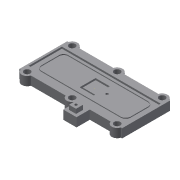
# Autodesk Inventor part: Bottom 6_12
Saved by Autodesk Inventor 2016 (Build 200138000, 138)
## iProperties
Created: 2015-05-18
Part Number: Bottom 6_12
Material: Generic
Document SubType Name: Modeling
Designer: Jonathan
Density: 1 g/cm^3
Appearance: Default
Author: Jonathan
Autodesk Inventor part; units mm, degrees
ref_plane "YZ Plane" through (0, 0, 0) normal (1, 0, 0) x (0, 1, 0)
ref_plane "XZ Plane" through (0, 0, 0) normal (0, 1, 0) x (-1, 0, 0)
ref_plane "XY Plane" through (0, 0, 0) normal (0, 0, 1) x (1, 0, 0)
sketch "Sketch1" plane through (0, 0, 0) normal (0, 1, 0) x (-1, 0, 0)
  line L0 (58, 27) -> (-58, 27)
  line L1 (-58, 27) -> (-58, -27)
  line L2 (-58, -27) -> (58, -27)
  line L3 (58, -27) -> (58, 27)
  line L4 (58, 27) -> (-58, -27) construction
  line L5 (-58, 27) -> (58, -27) construction
  point P0 (0, 0)
  dimension "d0" = 116
  dimension "d1" = 54
  constraints: 12 end point, 2 midpoint, 2 parallel, 1 horizontal, 1 perpendicular
  measures "d0" distance of L2.end L1.end
  measures "d1" distance of L2.end L0.start
extrude "Body" add sketch "Sketch1" along normal mid plane 10
sketch "Sketch2" plane through (0, 5, 0) normal (0, 1, 0) x (1, 0, 0)
  line L0 (-55.75, 18.75) -> (55.75, 18.75)
  line L1 (55.75, 18.75) -> (55.75, -18.75)
  line L2 (55.75, -18.75) -> (-55.75, -18.75)
  line L3 (-55.75, -18.75) -> (-55.75, 18.75)
  line L4 (-55.75, 18.75) -> (55.75, -18.75) construction
  line L5 (55.75, 18.75) -> (-55.75, -18.75) construction
  point P0 (0, 0)
  dimension "d4" = 111.5
  dimension "d5" = 37.5
  constraints: 12 end point, 2 midpoint, 2 parallel, 1 horizontal, 1 perpendicular
  measures "d4" distance of L1.end L2.end
  measures "d5" distance of L0.end L1.end
extrude "Top Socket" cut sketch "Sketch2" against normal blind 2
sketch "Sketch3" plane through (0, 3, 0) normal (0, 1, 0) x (1, 0, 0)
  line L0 (-8, -9) -> (8, -9)
  line L1 (8, -9) -> (8, 9)
  line L2 (8, 9) -> (-8, 9)
  line L3 (-8, 9) -> (-8, -9)
  line L4 (-8, -9) -> (8, 9) construction
  line L5 (8, -9) -> (-8, 9) construction
  point P0 (0, 0)
  dimension "d29" = 18
  dimension "d30" = 16
  constraints: 12 end point, 2 midpoint, 2 parallel, 1 horizontal, 1 perpendicular
  measures "d29" distance of L2.end L0.start
  measures "d30" distance of L1.end L2.end
extrude "Photoelectrode Bay" cut sketch "Sketch3" against normal blind 2
sketch "Sketch4" plane through (0, 3, 0) normal (0, 1, 0) x (1, 0, 0)
  circle A0 centre (14, 0) radius 1.45
  line L0 (-55.75, -18.75) -> (-55.75, 18.75) projected
  line L1 (-55.75, 0) -> (55.75, 0)
  line L2 (55.75, 18.75) -> (55.75, -18.75) projected
  line L3 (-55.75, -3) -> (55.75, -3)
  line L4 (8, 9) -> (8, -9) projected
  point P0 (0, 0)
  dimension "d11" = 2.9
  dimension "d20" = 3
  dimension "d97" = 6
  constraints: 4 end point, 2 midpoint, 2 point on line, 1 centre point, 1 parallel
  measures "d11" diameter of A0
  measures "d20" distance between parallel lines of L1 L3
  measures "d97" distance from line of A0.centre L4
revolve "Ref elec" cut sketch "Sketch4" angle 90 about axis through (-55.75, 3, 3) along (-1, 0, 0) contours L1 A0 | A0 L1
sketch "Sketch7" plane through (-58, 5, 27) normal (0, 0, 1) x (1, 0, 0)
  circle A0 centre (72, -5) radius 1.45
  circle A1 centre (72, -5) radius 1.45 projected
  point P0 (58, -5)
  dimension "d21" = 2.9
  constraints: 1 centre point, 1 concentric
  measures "d21" diameter of A0
extrude "Ref elec length" cut sketch "Sketch7" against normal up to surface (24 mm away)
sketch "Sketch8" plane through (-58, 5, 27) normal (0, 0, 1) x (1, 0, 0)
  line L0 (116, -10) -> (0, -10) projected
  line L1 (113.75, 0) -> (2.25, 0) projected
  line L2 (64.5, 0) -> (79.5, 0)
  line L3 (79.5, 0) -> (79.5, -10)
  line L4 (79.5, -10) -> (64.5, -10)
  line L5 (64.5, -10) -> (64.5, 0)
  line L6 (79.5, 0) -> (64.5, -10) construction
  line L7 (116, -10) -> (116, 0) projected
  point P0 (58, -5)
  point P1 (72, -5)
  point P2 (72, -10)
  dimension "d108" = 15
  dimension "d109" = 0
  constraints: 10 end point, 3 parallel, 1 horizontal, 1 midpoint, 1 perpendicular, 1 point on line
  measures "d108" distance between parallel lines of L3 L5
  measures "d109" distance between parallel lines of L1 L2
sketch "Sketch9" plane through (0, 1, 0) normal (0, 1, 0) x (1, 0, 0)
  line L0 (8, -9) -> (-8, -9) projected
  line L1 (8, -9) -> (-8, -9) projected
  line L2 (-8, -9) -> (8, -9)
  line L3 (8, -9) -> (8, -5.5)
  line L4 (8, -5.5) -> (-8, -5.5)
  line L5 (-8, -5.5) -> (-8, -9)
  dimension "d70" = 3.5
  constraints: 8 end point, 2 parallel, 1 horizontal, 1 perpendicular
  measures "d70" distance of L4.end L0.end
extrude "Photoelectrode Hole" cut sketch "Sketch9" against normal through all
sketch "Sketch12" plane through (0, 5, 0) normal (0, 1, 0) x (1, 0, 0)
  line L0 (58, 27) -> (-58, 27) projected
  circle A0 centre (-50.8, 25.4) radius 6
  line L1 (-58, -27) -> (-58, 27) projected
  line L2 (-58, 0) -> (58, 0)
  line L3 (58, 27) -> (58, -27) projected
  line L4 (-58, -27) -> (58, -27) projected
  line L5 (0, -27) -> (0, 27)
  circle A1 centre (50.8, 25.4) radius 6
  circle A2 centre (-50.8, -25.4) radius 6
  circle A3 centre (50.8, -25.4) radius 6
  line L6 (-50.8, 25.4) -> (50.8, 25.4)
  line L7 (-50.8, -25.4) -> (50.8, -25.4)
  circle A4 centre (0, 25.4) radius 6
  circle A5 centre (0, -25.4) radius 6
  point P0 (0, 0)
  dimension "d40" = 25.4
  dimension "d49" = 50.8
  dimension "d57" = 12
  constraints: 8 end point, 6 centre point, 5 midpoint, 4 symmetric about line, 1 equal radius, 1 horizontal, 1 parallel, 4 other
  measures "d40" distance from line of L6.start L2
  measures "d49" horizontal distance of L5.end L6.start
  measures "d57" diameter of A4
extrude "Screw clamp boss" add sketch "Sketch12" against normal up to surface (10 mm away) contours A1 L0 | L0 A1 | A4 L6 L5 L0 | L0 A4 | A5 L7 L5 | L5 L7 A5 | A4 L6 L5 | L5 L6 A4 | A3 L4 | L4 A3 | L5 L6 A4 L0 | L7 A5 L4 L5 | L5 L4 A5 L7 | A0 L0 | L0 A0 | A2 L4 | L4 A2 | L4 A5
sketch "Sketch15" plane through (0, 5, 0) normal (0, 1, 0) x (1, 0, 0)
  circle A0 centre (0, 25.4) radius 3.5
  arc A1 (5.7827, 27) -> (-5.7827, 27) centre (0, 25.4) ccw projected
  circle A2 centre (-50.8, 25.4) radius 3.5
  arc A3 (-45.0173, 27) -> (-56.5827, 27) centre (-50.8, 25.4) ccw projected
  line L0 (55.75, -18.75) -> (-55.75, -18.75) projected
  line L1 (0, -18.75) -> (0, 18.75)
  line L2 (-55.75, 18.75) -> (55.75, 18.75) projected
  line L3 (-58, 27) -> (-58, -27) projected
  line L4 (-58, 0) -> (58, 0)
  line L5 (58, -27) -> (58, 27) projected
  circle A4 centre (50.8, 25.4) radius 3.5
  circle A5 centre (0, -25.4) radius 3.5
  circle A6 centre (-50.8, -25.4) radius 3.5
  circle A7 centre (50.8, -25.4) radius 3.5
  point P0 (0, 0)
  dimension "d60" = 7
  constraints: 6 centre point, 4 end point, 4 midpoint, 4 symmetric about line, 2 concentric, 1 equal radius, 4 other
  measures "d60" diameter of A0
extrude "Screw Clamp Hole" cut sketch "Sketch15" against normal through all
sketch "Sketch18" plane through (-0.0162, 3, 0) normal (0, 1, 0) x (1, 0, 0)
  line L0 (-45, -15) -> (45, -15)
  line L1 (50, -10) -> (50, 10)
  line L2 (45, 15) -> (-45, 15)
  line L3 (-50, 10) -> (-50, -10)
  line L4 (-50, -15) -> (50, 15) construction
  line L5 (50, -15) -> (-50, 15) construction
  line L6 (-45, -15.5) -> (45, -15.5)
  line L7 (50.5, -10) -> (50.5, 10)
  line L8 (45, 15.5) -> (-45, 15.5)
  line L9 (-50.5, 10) -> (-50.5, -10)
  line L10 (-50.5, -15.5) -> (50.5, 15.5) construction
  line L11 (50.5, -15.5) -> (-50.5, 15.5) construction
  arc A0 (-50, -10) -> (-45, -15) centre (-45, -10) ccw
  arc A1 (45, -15) -> (50, -10) centre (45, -10) ccw
  arc A2 (50, 10) -> (45, 15) centre (45, 10) ccw
  arc A3 (-45, 15) -> (-50, 10) centre (-45, 10) ccw
  arc A4 (-50.5, -10) -> (-45, -15.5) centre (-45, -10) ccw
  arc A5 (45, -15.5) -> (50.5, -10) centre (45, -10) ccw
  arc A6 (50.5, 10) -> (45, 15.5) centre (45, 10) ccw
  arc A7 (-45, 15.5) -> (-50.5, 10) centre (-45, 10) ccw
  point P0 (0, 0)
  dimension "d83" = 100
  dimension "d84" = 30
  dimension "d85" = 0.5
  dimension "d86" = 0.5
  dimension "d87" = 5
  dimension "d88" = 5
  dimension "d89" = 5
  dimension "d90" = 5
  dimension "d91" = 5.5
  dimension "d92" = 5.5
  dimension "d93" = 5.5
  dimension "d94" = 5.5
  constraints: 24 end point, 16 point on circle, 16 point on line, 16 tangent, 8 centre point, 4 midpoint, 4 parallel, 2 horizontal, 2 perpendicular
  measures "d83" distance of L5.end L4.end
  measures "d84" distance of L4.end L5.start
  measures "d85" distance between parallel lines of L8 L2
  measures "d86" distance between parallel lines of L3 L9
  measures "d87" radius of A0
  measures "d88" radius of A1
  measures "d89" radius of A2
  measures "d90" radius of A3
  measures "d91" radius of A4
  measures "d92" radius of A5
  measures "d93" radius of A6
  measures "d94" radius of A7
extrude "Knife Edge" add sketch "Sketch18" along normal blind 1
extrude "Ref Electrode Outlet" add sketch "Sketch8" along normal blind 15
sketch "Sketch19" plane through (45.0173, -5, 27) normal (0, 0, 1) x (1, 0, 0)
  circle A0 centre (-31.0173, 5) radius 1.45
  circle A1 centre (-31.0173, 5) radius 1.45 projected
  line L0 (0, 10) -> (-39.2345, 10) projected
  line L1 (-29.5673, 10) -> (-18.6963, 10)
  line L2 (-23.5173, 10) -> (0, 10) projected
  point P0 (-45.0173, 5)
  constraints: 2 concentric, 2 end point, 2 point on line, 1 centre point
extrude "Extrusion22" cut sketch "Sketch19" along normal blind 9.5
sketch "Sketch20" plane through (0, 5, 0) normal (0, 1, 0) x (1, 0, 0)
  circle A0 centre (14, -35.05) radius 1.45
  circle A1 centre (14, 0) radius 1.45 projected
  line L0 (12.55, -36.5) -> (15.45, -36.5) projected
  point P0 (0, 0)
  constraints: 1 centre point, 1 equal radius, 1 tangent
extrude "Extrusion23" cut sketch "Sketch20" against normal blind 5 contours A0
sketch "Sketch21" plane through (0, 5, 0) normal (0, 1, 0) x (1, 0, 0)
  circle A0 centre (14, -35.05) radius 4
  circle A1 centre (14, -35.05) radius 1.45 projected
  line L0 (10, -39.05) -> (18, -39.05)
  line L1 (18, -39.05) -> (18, -31.05)
  line L2 (18, -31.05) -> (10, -31.05)
  line L3 (10, -31.05) -> (10, -39.05)
  line L4 (10, -39.05) -> (18, -31.05) construction
  line L5 (18, -39.05) -> (10, -31.05) construction
  point P0 (0, 0)
  dimension "d105" = 8
  constraints: 12 end point, 2 midpoint, 2 parallel, 2 tangent, 1 centre point, 1 concentric, 1 horizontal, 1 perpendicular
  measures "d105" diameter of A0
extrude "Extrusion24" add sketch "Sketch21" along normal blind 5
body "Solid1"
